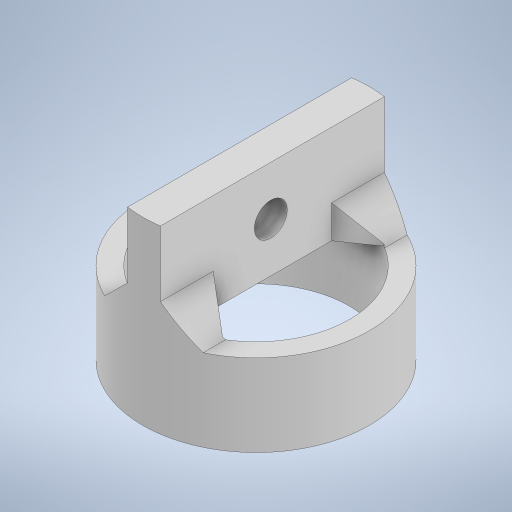
# Autodesk Inventor part: terminal_end_4.1mm_addon_new
Saved by Autodesk Inventor 2024 (Build 280153000, 153)
## iProperties
Created: 2024-04-25
Part Number: terminal_end_4.1mm_addon_new
Material: 일반
Document SubType Name: Modeling
Designer: Gihyeok Na
Density: 1 g/cm^3
Appearance: 기본값
Author: Gihyeok Na
Autodesk Inventor part; units mm, degrees
ref_plane "YZ Plane" through (0, 0, 0) normal (1, 0, 0) x (0, 1, 0)
ref_plane "XZ Plane" through (0, 0, 0) normal (0, 1, 0) x (-1, 0, 0)
ref_plane "XY Plane" through (0, 0, 0) normal (0, 0, 1) x (1, 0, 0)
sketch "스케치1" plane through (0, 0, 0) normal (0, 1, 0) x (-1, 0, 0)
  circle A0 centre (0, 0) radius 2.85
  circle A1 centre (0, 0) radius 3.45
  dimension "d0" = 5.7
  dimension "d1" = 6.9
  constraints: 2 centre point, 2 coincident
  measures "d0" diameter of A0
  measures "d1" diameter of A1
extrude "돌출1" add sketch "스케치1" along normal blind 2.5
sketch "스케치2" plane through (0, 2.5, 0) normal (0, 1, 0) x (1, 0, 0)
  circle A0 centre (0, 0) radius 3.45 projected
  circle A1 centre (0, 0) radius 3.45 projected
  line L0 (0.5, 3.4136) -> (-0.5, 3.4136)
  line L1 (-0.5, 3.4136) -> (-0.5, -3.4136)
  line L2 (-0.5, -3.4136) -> (0.5, -3.4136)
  line L3 (0.5, -3.4136) -> (0.5, 3.4136)
  line L4 (0.5, 3.4136) -> (-0.5, -3.4136) construction
  line L5 (-0.5, 3.4136) -> (0.5, -3.4136) construction
  point P0 (-0.5, -3.4136)
  point P1 (0.5, -3.4136)
  point P2 (0.5, 3.4136)
  point P3 (-0.5, 3.4136)
  dimension "d4" = 1
  constraints: 12 end point, 2 midpoint, 2 parallel, 1 horizontal, 1 perpendicular, 1 point on circle
  measures "d4" distance of L2.end L1.end
extrude "돌출2" add sketch "스케치2" along normal blind 3 contours L0 A0 | L3 L2 L1 L0 | A0 L2
chamfer "모따기1" distance 1 angle 45 4 edges at (0.5, 2.5, 3.1097) (0.5, 2.5, -3.1097) (-0.5, 2.5, -3.1097) (-0.5, 2.5, 3.1097)
chamfer "모따기2" distance 1 angle 45 4 edges at (-0.5, 3, -2.8058) (-0.5, 3, 2.8058) (0.5, 3, 2.8058) (0.5, 3, -2.8058)
sketch "스케치5" plane through (0.5, 5.5, 3.4136) normal (1, 0, 0) x (0, 0, -1)
  line L0 (5.2194, -2) -> (5.2194, -3) projected
  line L1 (6.8272, -2) -> (5.2194, -2) projected
  line L2 (6.8272, -2) -> (6.8272, 0) projected
  line L3 (0, 0) -> (6.8272, 0) projected
  line L4 (0, -2) -> (0, 0) projected
  line L5 (1.6078, -2) -> (0, -2) projected
  line L6 (1.6078, -3) -> (1.6078, -2) projected
  line L7 (1.6078, -3) -> (5.2194, -3) projected
  circle A0 centre (3.363, -1.5) radius 0.5
  line L8 (6.5204, -3) -> (0.3067, -3) projected
  point P0 (3.4136, -5.5)
  dimension "d15" = 1
  dimension "d16" = 1.5
  constraints: 1 centre point
  measures "d15" diameter of A0
  measures "d16" distance from line of L7 A0.centre
extrude "돌출4" cut sketch "스케치5" against normal blind 3 contours A0
